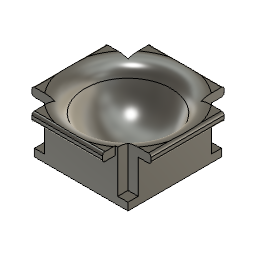
vessel_holder_bottom_500ml (Autodesk Fusion 360 design; units mm, degrees)
Autodesk Fusion 360 part; units mm, degrees
sketch "スケッチ1" plane through (0, 0, 0) normal (0, 0, 1) x (1, 0, 0)
  line L0 (55, -55) -> (-55, -55)
  line L1 (-55, -55) -> (-55, 55)
  line L2 (-55, 55) -> (55, 55)
  line L3 (55, 55) -> (55, -55)
  line L4 (55, -55) -> (-55, 55) construction
  line L5 (-55, -55) -> (55, 55) construction
  dimension "d1" = 110
  dimension "d2" = 110
  constraint horizontal L0
  constraint perpendicular L0 L1
  constraint parallel L0 L2
  constraint parallel L1 L3
  constraint coincident L4 origin
  constraint coincident L5 origin
  measures "d1" distance of L1.end L2.end
  measures "d2" distance of L0.end L1.end
extrude "押し出し1" add sketch "スケッチ1" along normal blind 59
sphere "球プリミティブ1" cut diameter 105 placed x (-1, 0, 0) y (0, -1, 0) z (0, 0, 1) at (0, 0, 59)
sketch "スケッチ9" plane through (0, 0, 59) normal (0, 0, 1) x (-1, 0, 0)
  circle A0 centre (0, 0) radius 52.5
  line L0 (-55, -55) -> (55, -55)
  line L1 (55, -55) -> (55, 55)
  line L2 (55, 55) -> (-55, 55)
  line L3 (-55, 55) -> (-55, -55)
  line L4 (-55, 55) -> (-43, 55)
  line L5 (-43, 55) -> (-43, 43)
  line L6 (-43, 43) -> (-55, 43)
  line L7 (-55, 43) -> (-55, 55)
  line L8 (55, -55) -> (43, -55)
  line L9 (43, -55) -> (43, -43)
  line L10 (43, -43) -> (55, -43)
  line L11 (55, -43) -> (55, -55)
  line L12 (-55, -55) -> (-43, -55)
  line L13 (-43, -55) -> (-43, -43)
  line L14 (-43, -43) -> (-55, -43)
  line L15 (-55, -43) -> (-55, -55)
  line L16 (55, 55) -> (43, 55)
  line L17 (43, 55) -> (43, 43)
  line L18 (43, 43) -> (55, 43)
  line L19 (55, 43) -> (55, 55)
  dimension "d18" = 12
  dimension "d19" = 12
  dimension "d20" = 12
  dimension "d21" = 12
  dimension "d22" = 12
  dimension "d23" = 12
  dimension "d24" = 12
  dimension "d25" = 12
  constraint horizontal L4
  constraint vertical L5
  constraint horizontal L6
  constraint vertical L7
  constraint coincident L2.end L3.start
  constraint horizontal L8
  constraint vertical L9
  constraint horizontal L10
  constraint vertical L11
  constraint coincident L0.end L1.start
  constraint horizontal L12
  constraint vertical L13
  constraint horizontal L14
  constraint vertical L15
  constraint coincident L0.start L3.end
  constraint horizontal L16
  constraint vertical L17
  constraint horizontal L18
  constraint vertical L19
  constraint coincident L1.end L2.start
  measures "d18" distance of L2.end L4.end
  measures "d19" distance of L2.end L6.end
  measures "d20" distance of L0.end L8.end
  measures "d21" distance of L0.end L10.end
  measures "d22" distance of L0.start L12.end
  measures "d23" distance of L0.start L14.end
  measures "d24" distance of L1.end L16.end
  measures "d25" distance of L1.end L18.end
extrude "押し出し6" cut sketch "スケッチ9" against normal blind 50 contours L0 L3 L12 L13 L14 L15 | L0 L1 L8 L9 L10 L11 | L2 L3 L4 L5 L6 L7 | L1 L2 L16 L17 L18 L19
sketch "スケッチ10" plane through (0, -55, 0) normal (0, -1, 0) x (1, 0, 0)
  line L0 (-43, 59) -> (-43, 9)
  line L1 (-43, 9) -> (-55, 9)
  line L2 (-55, 9) -> (-55, 0)
  line L3 (-55, 0) -> (55, 0)
  line L4 (55, 0) -> (55, 9)
  line L5 (55, 9) -> (43, 9)
  line L6 (43, 9) -> (43, 59)
  line L7 (43, 59) -> (-43, 59)
  line L8 (-43, 59) -> (40, 59)
  line L9 (40, 59) -> (40, 49)
  line L10 (40, 49) -> (-43, 49)
  line L11 (-43, 49) -> (-43, 59)
  dimension "d28" = 10
  constraint horizontal L8
  constraint vertical L9
  constraint horizontal L10
  constraint vertical L11
  constraint coincident L0.start L7.end
  measures "d28" distance of L0.start L10.end
sketch "スケッチ11" plane through (55, 0, 0) normal (1, 0, 0) x (0, 1, 0)
  line L0 (55, 9) -> (43, 9)
  line L1 (43, 9) -> (43, 59)
  line L2 (43, 59) -> (-43, 59)
  line L3 (-43, 59) -> (-43, 9)
  line L4 (-43, 9) -> (-55, 9)
  line L5 (-55, 9) -> (-55, 0)
  line L6 (-55, 0) -> (55, 0)
  line L7 (55, 0) -> (55, 9)
  line L8 (-43, 59) -> (43, 59)
  line L9 (43, 59) -> (43, 48.8532)
  line L10 (43, 48.8532) -> (-43, 48.8532)
  line L11 (-43, 48.8532) -> (-43, 59)
  constraint horizontal L8
  constraint vertical L9
  constraint horizontal L10
  constraint vertical L11
  constraint coincident L1 L9.end
  constraint coincident L2.end L3.start
sketch "スケッチ12" plane through (0, 55, 0) normal (0, 1, 0) x (-1, 0, 0)
  line L0 (43, 9) -> (43, 59)
  line L1 (43, 59) -> (-43, 59)
  line L2 (-43, 59) -> (-43, 9)
  line L3 (-43, 9) -> (-55, 9)
  line L4 (-55, 9) -> (-55, 0)
  line L5 (-55, 0) -> (55, 0)
  line L6 (55, 0) -> (55, 9)
  line L7 (55, 9) -> (43, 9)
  line L8 (-43, 59) -> (43, 59)
  line L9 (43, 59) -> (43, 48.8532)
  line L10 (43, 48.8532) -> (-43, 48.8532)
  line L11 (-43, 48.8532) -> (-43, 59)
  constraint horizontal L8
  constraint vertical L9
  constraint horizontal L10
  constraint vertical L11
  constraint coincident L0 L9.end
  constraint coincident L1.end L2.start
sketch "スケッチ13" plane through (-55, 0, 0) normal (-1, 0, 0) x (0, -1, 0)
  line L0 (-43, 59) -> (-43, 9)
  line L1 (-43, 9) -> (-55, 9)
  line L2 (-55, 9) -> (-55, 0)
  line L3 (-55, 0) -> (55, 0)
  line L4 (55, 0) -> (55, 9)
  line L5 (55, 9) -> (43, 9)
  line L6 (43, 9) -> (43, 59)
  line L7 (43, 59) -> (-43, 59)
  line L8 (-43, 59) -> (43, 59)
  line L9 (43, 59) -> (43, 48.8532)
  line L10 (43, 48.8532) -> (-43, 48.8532)
  line L11 (-43, 48.8532) -> (-43, 59)
  constraint horizontal L8
  constraint vertical L9
  constraint horizontal L10
  constraint vertical L11
  constraint coincident L6 L9.end
  constraint coincident L0.start L7.end
extrude "押し出し7" add sketch "スケッチ13" along normal blind 15 contours L0 L6 L7 L8 L9 L10 L11
extrude "押し出し8" add sketch "スケッチ12" along normal blind 15 contours L0 L1 L2 L8 L9 L10 L11
extrude "押し出し9" add sketch "スケッチ10" along normal blind 15 contours L0 L7 L8 L9 L10 L11
extrude "押し出し10" add sketch "スケッチ11" along normal blind 15 contours L1 L2 L3 L8 L9 L10 L11
fillet "フィレット2" radius 20 1 edges at (-18.9848, -48.9472, 59)
fillet "フィレット3" radius 3 4 edges at (-1.5, -70, 59) (70, 0, 59) (0, 70, 59) (-70, 0, 59)
fillet "フィレット4" radius 3 4 edges at (-1.5, -70, 49) (70, 0, 48.8532) (0, 70, 48.8532) (-70, 0, 48.8532)
sketch "スケッチ3" plane through (55, 0, 0) normal (1, 0, 0) x (0, 1, 0)
  line L0 (-55, 0) -> (55, 0)
  line L1 (55, 0) -> (55, 59)
  line L2 (55, 59) -> (-55, 59)
  line L3 (-55, 59) -> (-55, 0)
  line L4 (-55, 9.8951) -> (55, 9.8951)
  line L5 (55, 9.8951) -> (55, 0)
  line L6 (55, 0) -> (-55, 0)
  line L7 (-55, 0) -> (-55, 9.8951)
  constraint horizontal L4
  constraint vertical L5
  constraint horizontal L6
  constraint vertical L7
  constraint coincident L0.end L1.start
  constraint coincident L3 L4.start
extrude "押し出し2" [suppressed]
sketch "スケッチ4" plane through (-55, 0, 0) normal (-1, 0, 0) x (0, -1, 0)
  line L0 (-55, 0) -> (55, 0)
  line L1 (55, 0) -> (55, 59)
  line L2 (55, 59) -> (-55, 59)
  line L3 (-55, 59) -> (-55, 0)
  line L4 (-55, 9.8951) -> (55, 9.8951)
  line L5 (55, 9.8951) -> (55, 0)
  line L6 (55, 0) -> (-55, 0)
  line L7 (-55, 0) -> (-55, 9.8951)
  constraint horizontal L4
  constraint vertical L5
  constraint horizontal L6
  constraint vertical L7
  constraint coincident L0.end L1.start
  constraint coincident L3 L4.start
extrude "押し出し3" [suppressed]
sketch "スケッチ8" plane through (0, 0, 59) normal (0, 0, 1) x (-1, 0, 0)
  circle A0 centre (0, 0) radius 52.5
  line L0 (-55, -55) -> (55, -55)
  line L1 (55, -55) -> (55, 55)
  line L2 (55, 55) -> (-55, 55)
  line L3 (-55, 55) -> (-55, -55)
  line L4 (55, -55) -> (40, -55)
  line L5 (40, -55) -> (40, -40)
  line L6 (40, -40) -> (55, -40)
  line L7 (55, -40) -> (55, -55)
  dimension "d16" = 15
  dimension "d17" = 15
  constraint horizontal L4
  constraint vertical L5
  constraint horizontal L6
  constraint vertical L7
  constraint coincident L0.end L1.start
  measures "d16" distance of L0.end L4.end
  measures "d17" distance of L0.end L6.end
sketch "スケッチ6" plane through (0, -55, 0) normal (0, -1, 0) x (1, 0, 0)
  line L0 (-75, 0) -> (75, 0)
  line L1 (75, 0) -> (75, 9.8951)
  line L2 (75, 9.8951) -> (55, 9.8951)
  line L3 (55, 9.8951) -> (55, 59)
  line L4 (55, 59) -> (-55, 59)
  line L5 (-55, 59) -> (-55, 9.8951)
  line L6 (-55, 9.8951) -> (-75, 9.8951)
  line L7 (-75, 9.8951) -> (-75, 0)
  line L8 (-55, 59) -> (55, 59)
  line L9 (55, 59) -> (55, 50)
  line L10 (55, 50) -> (-55, 50)
  line L11 (-55, 50) -> (-55, 59)
  constraint horizontal L8
  constraint vertical L9
  constraint horizontal L10
  constraint vertical L11
  constraint coincident L3 L9.end
  constraint coincident L4.end L5.start
extrude "押し出し4" [suppressed]
sketch "スケッチ7" plane through (0, 55, 0) normal (0, 1, 0) x (-1, 0, 0)
  line L0 (-75, 0) -> (75, 0)
  line L1 (75, 0) -> (75, 9.8951)
  line L2 (75, 9.8951) -> (55, 9.8951)
  line L3 (55, 9.8951) -> (55, 59)
  line L4 (55, 59) -> (-55, 59)
  line L5 (-55, 59) -> (-55, 9.8951)
  line L6 (-55, 9.8951) -> (-75, 9.8951)
  line L7 (-75, 9.8951) -> (-75, 0)
  line L8 (-55, 59) -> (55, 59)
  line L9 (55, 59) -> (55, 50)
  line L10 (55, 50) -> (-55, 50)
  line L11 (-55, 50) -> (-55, 59)
  constraint horizontal L8
  constraint vertical L9
  constraint horizontal L10
  constraint vertical L11
  constraint coincident L3 L9.end
  constraint coincident L4.end L5.start
extrude "押し出し5" [suppressed]
fillet "フィレット1" [suppressed]
